Autodesk Inventor part; units mm, degrees
(part 5 of 6)
  line L1245 (-76.5118, -134.1228) -> (-98.4236, -156.0346) projected
  line L1246 (-98.4236, -156.0346) -> (-76.5118, -177.9464) projected
  line L1247 (-76.5118, -177.9464) -> (-54.6, -156.0346) projected
  line L1248 (72.9197, -181.5385) -> (51.0079, -159.6267) projected
  line L1249 (51.0079, -159.6267) -> (29.096, -181.5385) projected
  line L1250 (29.096, -181.5385) -> (51.0079, -203.4504) projected
  line L1251 (51.0079, -203.4504) -> (72.9197, -181.5385) projected
  line L1252 (-72.9197, -130.5307) -> (-51.0079, -152.4425) projected
  line L1253 (-51.0079, -152.4425) -> (-29.096, -130.5307) projected
  line L1254 (-29.096, -130.5307) -> (-51.0079, -108.6189) projected
  line L1255 (-51.0079, -108.6189) -> (-72.9197, -130.5307) projected
  line L1256 (-146.05, -222.25) -> (-146.05, -247.4846) projected
  line L1257 (-146.05, -247.4846) -> (-131.1117, -232.5464) projected
  line L1258 (-131.1117, -232.5464) -> (-146.2009, -217.4573) projected
  arc A181 (-146.05, -222.25) -> (-146.2009, -217.4573) centre (-222.25, -222.25) ccw projected
  line L1259 (-29.096, -232.5464) -> (-51.0079, -210.6346) projected
  line L1260 (-51.0079, -210.6346) -> (-72.9197, -232.5464) projected
  line L1261 (-72.9197, -232.5464) -> (-51.0079, -254.4582) projected
  line L1262 (-51.0079, -254.4582) -> (-29.096, -232.5464) projected
  line L1263 (-43.9918, -298.45) -> (-29.096, -283.5542) projected
  line L1264 (-29.096, -283.5542) -> (-51.0079, -261.6424) projected
  line L1265 (-51.0079, -261.6424) -> (-72.9197, -283.5542) projected
  line L1266 (-72.9197, -283.5542) -> (-58.0239, -298.45) projected
  line L1267 (-58.0239, -298.45) -> (-43.9918, -298.45) projected
  line L1268 (-87.8154, -298.45) -> (-65.2081, -298.45) projected
  line L1269 (-65.2081, -298.45) -> (-76.5118, -287.1463) projected
  line L1270 (-76.5118, -287.1463) -> (-87.8154, -298.45) projected
  line L1271 (80.1039, -283.5542) -> (94.9996, -298.45) projected
  line L1272 (94.9996, -298.45) -> (109.0318, -298.45) projected
  line L1273 (109.0318, -298.45) -> (123.9275, -283.5542) projected
  line L1274 (123.9275, -283.5542) -> (102.0157, -261.6424) projected
  line L1275 (102.0157, -261.6424) -> (80.1039, -283.5542) projected
  line L1276 (14.2003, -298.45) -> (36.8076, -298.45) projected
  line L1277 (36.8076, -298.45) -> (25.5039, -287.1463) projected
  line L1278 (25.5039, -287.1463) -> (14.2003, -298.45) projected
  line L1279 (80.1039, -181.5385) -> (102.0157, -203.4504) projected
  line L1280 (102.0157, -203.4504) -> (123.9275, -181.5385) projected
  line L1281 (123.9275, -181.5385) -> (102.0157, -159.6267) projected
  line L1282 (102.0157, -159.6267) -> (80.1039, -181.5385) projected
  line L1283 (225.9432, -79.5228) -> (204.0314, -57.611) projected
  line L1284 (204.0314, -57.611) -> (182.1196, -79.5228) projected
  line L1285 (182.1196, -79.5228) -> (204.0314, -101.4346) projected
  line L1286 (204.0314, -101.4346) -> (225.9432, -79.5228) projected
  line L1287 (298.45, -14.2003) -> (284.1353, -28.515) projected
  line L1288 (284.1353, -28.515) -> (298.45, -42.8297) projected
  line L1289 (298.45, -42.8297) -> (298.45, -14.2003) projected
  line L1290 (258.6314, -54.0189) -> (280.5432, -75.9307) projected
  line L1291 (280.5432, -75.9307) -> (298.45, -58.0239) projected
  line L1292 (298.45, -58.0239) -> (298.45, -50.0139) projected
  line L1293 (298.45, -50.0139) -> (280.5432, -32.1071) projected
  line L1294 (280.5432, -32.1071) -> (258.6314, -54.0189) projected
  arc A182 (222.25, -146.05) -> (217.4573, -146.2009) centre (222.25, -222.25) ccw projected
  line L1295 (222.25, -146.05) -> (241.4626, -146.05) projected
  line L1296 (241.4626, -146.05) -> (229.5353, -134.1228) projected
  line L1297 (229.5353, -134.1228) -> (217.4573, -146.2009) projected
  line L1298 (131.1117, -181.5385) -> (149.4183, -199.8451) projected
  arc A183 (165.1681, -171.7713) -> (149.4183, -199.8451) centre (222.25, -222.25) ccw projected
  line L1299 (165.1681, -171.7713) -> (153.0236, -159.6267) projected
  line L1300 (153.0236, -159.6267) -> (131.1117, -181.5385) projected
  line L1301 (7.0161, -298.45) -> (21.9118, -283.5542) projected
  line L1302 (21.9118, -283.5542) -> (0, -261.6424) projected
  line L1303 (0, -261.6424) -> (-21.9118, -283.5542) projected
  line L1304 (-21.9118, -283.5542) -> (-7.0161, -298.45) projected
  line L1305 (-7.0161, -298.45) -> (7.0161, -298.45) projected
  line L1306 (298.45, 138.8233) -> (284.1353, 124.5086) projected
  line L1307 (284.1353, 124.5086) -> (298.45, 110.1939) projected
  line L1308 (298.45, 110.1939) -> (298.45, 138.8233) projected
  line L1309 (258.6314, 99.0047) -> (280.5432, 77.0928) projected
  line L1310 (280.5432, 77.0928) -> (298.45, 94.9996) projected
  line L1311 (298.45, 94.9996) -> (298.45, 103.0097) projected
  line L1312 (298.45, 103.0097) -> (280.5432, 120.9165) projected
  line L1313 (280.5432, 120.9165) -> (258.6314, 99.0047) projected
  line L1314 (233.1274, 22.4929) -> (255.0393, 0.5811) projected
  line L1315 (255.0393, 0.5811) -> (276.9511, 22.4929) projected
  line L1316 (276.9511, 22.4929) -> (255.0393, 44.4047) projected
  line L1317 (255.0393, 44.4047) -> (233.1274, 22.4929) projected
  line L1318 (207.6235, -3.011) -> (229.5353, -24.9229) projected
  line L1319 (229.5353, -24.9229) -> (251.4472, -3.011) projected
  line L1320 (251.4472, -3.011) -> (229.5353, 18.9008) projected
  line L1321 (229.5353, 18.9008) -> (207.6235, -3.011) projected
  line L1322 (174.9354, -28.515) -> (153.0236, -6.6031) projected
  line L1323 (153.0236, -6.6031) -> (131.1117, -28.515) projected
  line L1324 (131.1117, -28.515) -> (153.0236, -50.4268) projected
  line L1325 (153.0236, -50.4268) -> (174.9354, -28.515) projected
  line L1326 (159.5933, 7.1508) -> (174.933, 22.4952) projected
  line L1327 (174.933, 22.4952) -> (153.0236, 44.4047) projected
  line L1328 (153.0236, 44.4047) -> (131.1117, 22.4929) projected
  line L1329 (131.1117, 22.4929) -> (153.0236, 0.5811) projected
  line L1330 (153.0236, 0.5811) -> (159.5933, 7.1508) projected
  line L1331 (149.4315, 47.9968) -> (127.5196, 69.9086) projected
  line L1332 (127.5196, 69.9086) -> (105.6078, 47.9968) projected
  line L1333 (105.6078, 47.9968) -> (127.5196, 26.085) projected
  line L1334 (127.5196, 26.085) -> (149.4315, 47.9968) projected
  line L1335 (156.6157, 99.0047) -> (178.5275, 77.0928) projected
  line L1336 (178.5275, 77.0928) -> (200.4393, 99.0047) projected
  line L1337 (200.4393, 99.0047) -> (178.5275, 120.9165) projected
  line L1338 (178.5275, 120.9165) -> (156.6157, 99.0047) projected
  line L1339 (80.1039, 175.5165) -> (102.0157, 153.6046) projected
  line L1340 (102.0157, 153.6046) -> (123.9275, 175.5165) projected
  line L1341 (123.9275, 175.5165) -> (102.0157, 197.4283) projected
  line L1342 (102.0157, 197.4283) -> (80.1039, 175.5165) projected
  line L1343 (0, 146.4204) -> (-21.9118, 124.5086) projected
  line L1344 (-21.9118, 124.5086) -> (0, 102.5968) projected
  line L1345 (0, 102.5968) -> (21.9118, 124.5086) projected
  line L1346 (21.9118, 124.5086) -> (0, 146.4204) projected
  line L1347 (146.05, 222.25) -> (146.05, 241.4626) projected
  line L1348 (146.05, 241.4626) -> (131.1117, 226.5243) projected
  line L1349 (131.1117, 226.5243) -> (146.9294, 210.7066) projected
  arc A184 (146.05, 222.25) -> (146.9294, 210.7066) centre (222.25, 222.25) ccw projected
  line L1350 (80.1039, -130.5307) -> (102.0157, -152.4425) projected
  line L1351 (102.0157, -152.4425) -> (123.9275, -130.5307) projected
  line L1352 (123.9275, -130.5307) -> (102.0157, -108.6189) projected
  line L1353 (102.0157, -108.6189) -> (80.1039, -130.5307) projected
  line L1354 (47.4158, -156.0346) -> (25.5039, -134.1228) projected
  line L1355 (25.5039, -134.1228) -> (3.5921, -156.0346) projected
  line L1356 (3.5921, -156.0346) -> (25.5039, -177.9464) projected
  line L1357 (25.5039, -177.9464) -> (47.4158, -156.0346) projected
  line L1358 (98.4236, 252.0282) -> (76.5118, 273.9401) projected
  line L1359 (76.5118, 273.9401) -> (54.6, 252.0282) projected
  line L1360 (54.6, 252.0282) -> (76.5118, 230.1164) projected
  line L1361 (76.5118, 230.1164) -> (98.4236, 252.0282) projected
  line L1362 (3.5921, 252.0282) -> (25.5039, 230.1164) projected
  line L1363 (25.5039, 230.1164) -> (47.4158, 252.0282) projected
  line L1364 (47.4158, 252.0282) -> (25.5039, 273.9401) projected
  line L1365 (25.5039, 273.9401) -> (3.5921, 252.0282) projected
  line L1366 (-3.5921, 252.0282) -> (-25.5039, 273.9401) projected
  line L1367 (-25.5039, 273.9401) -> (-47.4158, 252.0282) projected
  line L1368 (-47.4158, 252.0282) -> (-25.5039, 230.1164) projected
  line L1369 (-25.5039, 230.1164) -> (-3.5921, 252.0282) projected
  line L1370 (-103.0097, 298.45) -> (-123.9275, 277.5322) projected
  line L1371 (-123.9275, 277.5322) -> (-102.0157, 255.6203) projected
  line L1372 (-102.0157, 255.6203) -> (-80.1039, 277.5322) projected
  line L1373 (-80.1039, 277.5322) -> (-101.0217, 298.45) projected
  line L1374 (-101.0217, 298.45) -> (-103.0097, 298.45) projected
  line L1375 (-80.1039, 226.5243) -> (-102.0157, 248.4361) projected
  line L1376 (-102.0157, 248.4361) -> (-123.9275, 226.5243) projected
  line L1377 (-123.9275, 226.5243) -> (-102.0157, 204.6125) projected
  line L1378 (-102.0157, 204.6125) -> (-80.1039, 226.5243) projected
  line L1379 (-105.6078, 201.0204) -> (-127.5196, 222.9322) projected
  line L1380 (-127.5196, 222.9322) -> (-148.9209, 201.531) projected
  arc A185 (-149.1495, 200.7384) -> (-148.9209, 201.531) centre (-222.25, 222.25) ccw projected
  line L1381 (-149.1495, 200.7384) -> (-127.5196, 179.1086) projected
  line L1382 (-127.5196, 179.1086) -> (-105.6078, 201.0204) projected
  line L1383 (-80.1039, 175.5165) -> (-102.0157, 197.4283) projected
  line L1384 (-102.0157, 197.4283) -> (-123.9275, 175.5165) projected
  line L1385 (-123.9275, 175.5165) -> (-102.0157, 153.6046) projected
  line L1386 (-102.0157, 153.6046) -> (-80.1039, 175.5165) projected
  line L1387 (-3.5921, 150.0125) -> (-25.5039, 171.9243) projected
  line L1388 (-25.5039, 171.9243) -> (-47.4158, 150.0125) projected
  line L1389 (-47.4158, 150.0125) -> (-25.5039, 128.1007) projected
  line L1390 (-25.5039, 128.1007) -> (-3.5921, 150.0125) projected
  line L1391 (-131.1117, 124.5086) -> (-153.0236, 146.4204) projected
  line L1392 (-153.0236, 146.4204) -> (-174.9354, 124.5086) projected
  line L1393 (-174.9354, 124.5086) -> (-153.0236, 102.5968) projected
  line L1394 (-153.0236, 102.5968) -> (-131.1117, 124.5086) projected
  line L1395 (-131.1117, 73.5007) -> (-153.0236, 95.4126) projected
  line L1396 (-153.0236, 95.4126) -> (-174.9354, 73.5007) projected
  line L1397 (-174.9354, 73.5007) -> (-153.0236, 51.5889) projected
  line L1398 (-153.0236, 51.5889) -> (-131.1117, 73.5007) projected
  line L1399 (-149.4315, -54.0189) -> (-127.5196, -75.9307) projected
  line L1400 (-127.5196, -75.9307) -> (-105.6078, -54.0189) projected
  line L1401 (-105.6078, -54.0189) -> (-127.5196, -32.1071) projected
  line L1402 (-127.5196, -32.1071) -> (-149.4315, -54.0189) projected
  line L1403 (-131.1117, -79.5228) -> (-153.0236, -57.611) projected
  line L1404 (-153.0236, -57.611) -> (-174.9354, -79.5228) projected
  line L1405 (-174.9354, -79.5228) -> (-153.0236, -101.4346) projected
  line L1406 (-153.0236, -101.4346) -> (-131.1117, -79.5228) projected
  arc A186 (-222.25, 146.05) -> (-210.7066, 146.9294) centre (-222.25, 222.25) ccw projected
  line L1407 (-222.25, 146.05) -> (-247.4846, 146.05) projected
  line L1408 (-247.4846, 146.05) -> (-229.5353, 128.1007) projected
  line L1409 (-229.5353, 128.1007) -> (-210.7066, 146.9294) projected
  line L1410 (-258.6314, 99.0047) -> (-280.5432, 120.9165) projected
  line L1411 (-280.5432, 120.9165) -> (-298.45, 103.0097) projected
  line L1412 (-298.45, 103.0097) -> (-298.45, 94.9996) projected
  line L1413 (-298.45, 94.9996) -> (-280.5432, 77.0928) projected
  line L1414 (-280.5432, 77.0928) -> (-258.6314, 99.0047) projected
  line L1415 (-156.6157, 47.9968) -> (-178.5275, 69.9086) projected
  line L1416 (-178.5275, 69.9086) -> (-200.4331, 48.0031) projected
  line L1417 (-200.4331, 48.0031) -> (-178.5246, 26.0879) projected
  line L1418 (-178.5246, 26.0879) -> (-156.6157, 47.9968) projected
  line L1419 (-258.6314, 47.9968) -> (-280.5432, 69.9086) projected
  line L1420 (-280.5432, 69.9086) -> (-298.45, 52.0018) projected
  line L1421 (-298.45, 52.0018) -> (-298.45, 43.9918) projected
  line L1422 (-298.45, 43.9918) -> (-280.5432, 26.085) projected
  line L1423 (-280.5432, 26.085) -> (-258.6314, 47.9968) projected
  line L1424 (-233.1274, -28.515) -> (-255.0393, -6.6031) projected
  line L1425 (-255.0393, -6.6031) -> (-276.9511, -28.515) projected
  line L1426 (-276.9511, -28.515) -> (-255.0393, -50.4268) projected
  line L1427 (-255.0393, -50.4268) -> (-233.1274, -28.515) projected
  line L1428 (-298.45, -42.8297) -> (-284.1353, -28.515) projected
  line L1429 (-284.1353, -28.515) -> (-298.45, -14.2003) projected
  line L1430 (-298.45, -14.2003) -> (-298.45, -42.8297) projected
  line L1431 (-298.45, -93.8375) -> (-284.1353, -79.5228) projected
  line L1432 (-284.1353, -79.5228) -> (-298.45, -65.2081) projected
  line L1433 (-298.45, -65.2081) -> (-298.45, -93.8375) projected
  line L1434 (-178.5275, 18.9008) -> (-200.4393, -3.011) projected
  line L1435 (-200.4393, -3.011) -> (-178.5275, -24.9229) projected
  line L1436 (-178.5275, -24.9229) -> (-156.6157, -3.011) projected
  line L1437 (-156.6157, -3.011) -> (-178.5275, 18.9008) projected
  line L1438 (-258.6314, -3.011) -> (-280.5432, 18.9008) projected
  line L1439 (-280.5432, 18.9008) -> (-298.45, 0.994) projected
  line L1440 (-298.45, 0.994) -> (-298.45, -7.0161) projected
  line L1441 (-298.45, -7.0161) -> (-280.5432, -24.9229) projected
  line L1442 (-280.5432, -24.9229) -> (-258.6314, -3.011) projected
  line L1443 (-233.1274, 22.4929) -> (-255.0393, 44.4047) projected
  line L1444 (-255.0393, 44.4047) -> (-276.9511, 22.4929) projected
  line L1445 (-276.9511, 22.4929) -> (-255.0393, 0.5811) projected
  line L1446 (-255.0393, 0.5811) -> (-233.1274, 22.4929) projected
  line L1447 (-182.1196, 73.5007) -> (-204.0314, 95.4126) projected
  line L1448 (-204.0314, 95.4126) -> (-225.9331, 73.5109) projected
  line L1449 (-225.9331, 73.5109) -> (-204.0246, 51.5957) projected
  line L1450 (-204.0246, 51.5957) -> (-182.1196, 73.5007) projected
  line L1451 (-298.45, 110.1939) -> (-284.1353, 124.5086) projected
  line L1452 (-284.1353, 124.5086) -> (-298.45, 138.8233) projected
  line L1453 (-298.45, 138.8233) -> (-298.45, 110.1939) projected
  line L1454 (-21.9118, 175.5165) -> (0, 153.6046) projected
  line L1455 (0, 153.6046) -> (21.9118, 175.5165) projected
  line L1456 (21.9118, 175.5165) -> (0, 197.4283) projected
  line L1457 (0, 197.4283) -> (-21.9118, 175.5165) projected
  line L1458 (-105.6078, -105.0267) -> (-127.5196, -83.1149) projected
  line L1459 (-127.5196, -83.1149) -> (-149.4315, -105.0267) projected
  line L1460 (-149.4315, -105.0267) -> (-127.5196, -126.9386) projected
  line L1461 (-127.5196, -126.9386) -> (-105.6078, -105.0267) projected
  line L1462 (-153.0236, -50.4268) -> (-131.1117, -28.515) projected
  line L1463 (-131.1117, -28.515) -> (-153.0236, -6.6031) projected
  line L1464 (-153.0236, -6.6031) -> (-174.9354, -28.515) projected
  line L1465 (-174.9354, -28.515) -> (-153.0236, -50.4268) projected
  line L1466 (-156.6157, 99.0047) -> (-178.5275, 120.9165) projected
  line L1467 (-178.5275, 120.9165) -> (-200.4393, 99.0047) projected
  line L1468 (-200.4393, 99.0047) -> (-178.5275, 77.0928) projected
  line L1469 (-178.5275, 77.0928) -> (-156.6157, 99.0047) projected
  line L1470 (-105.6078, 99.0047) -> (-127.5196, 120.9165) projected
  line L1471 (-127.5196, 120.9165) -> (-149.4315, 99.0047) projected
  line L1472 (-149.4315, 99.0047) -> (-127.5196, 77.0928) projected
  line L1473 (-127.5196, 77.0928) -> (-105.6078, 99.0047) projected
  line L1474 (-29.096, 175.5165) -> (-51.0079, 197.4283) projected
  line L1475 (-51.0079, 197.4283) -> (-72.9197, 175.5165) projected
  line L1476 (-72.9197, 175.5165) -> (-51.0079, 153.6046) projected
  line L1477 (-51.0079, 153.6046) -> (-29.096, 175.5165) projected
  line L1478 (-149.4315, 150.0125) -> (-127.5196, 128.1007) projected
  line L1479 (-127.5196, 128.1007) -> (-105.6078, 150.0125) projected
  line L1480 (-105.6078, 150.0125) -> (-127.5196, 171.9243) projected
  line L1481 (-127.5196, 171.9243) -> (-149.4315, 150.0125) projected
  line L1482 (-54.6, 201.0204) -> (-76.5118, 222.9322) projected
  line L1483 (-76.5118, 222.9322) -> (-98.4236, 201.0204) projected
  line L1484 (-98.4236, 201.0204) -> (-76.5118, 179.1086) projected
  line L1485 (-76.5118, 179.1086) -> (-54.6, 201.0204) projected
  line L1486 (-105.6078, 252.0282) -> (-127.5196, 273.9401) projected
  line L1487 (-127.5196, 273.9401) -> (-146.05, 255.4097) projected
  line L1488 (-146.05, 255.4097) -> (-146.05, 248.6468) projected
  line L1489 (-146.05, 248.6468) -> (-127.5196, 230.1164) projected
  line L1490 (-127.5196, 230.1164) -> (-105.6078, 252.0282) projected
  line L1491 (-59.186, 298.45) -> (-93.8375, 298.45) projected
  line L1492 (-93.8375, 298.45) -> (-76.5118, 281.1243) projected
  line L1493 (-76.5118, 281.1243) -> (-59.186, 298.45) projected
  line L1494 (21.9118, 226.5243) -> (0, 248.4361) projected
  line L1495 (0, 248.4361) -> (-21.9118, 226.5243) projected
  line L1496 (-21.9118, 226.5243) -> (0, 204.6125) projected
  line L1497 (0, 204.6125) -> (21.9118, 226.5243) projected
  line L1498 (29.096, 226.5243) -> (51.0079, 204.6125) projected
  line L1499 (51.0079, 204.6125) -> (72.9197, 226.5243) projected
  line L1500 (72.9197, 226.5243) -> (51.0079, 248.4361) projected
  line L1501 (51.0079, 248.4361) -> (29.096, 226.5243) projected
  line L1502 (103.0097, 298.45) -> (101.0217, 298.45) projected
  line L1503 (101.0217, 298.45) -> (80.1039, 277.5322) projected
  line L1504 (80.1039, 277.5322) -> (102.0157, 255.6203) projected
  line L1505 (102.0157, 255.6203) -> (123.9275, 277.5322) projected
  line L1506 (123.9275, 277.5322) -> (103.0097, 298.45) projected
  line L1507 (29.096, -130.5307) -> (51.0079, -152.4425) projected
  line L1508 (51.0079, -152.4425) -> (72.9197, -130.5307) projected
  line L1509 (72.9197, -130.5307) -> (51.0079, -108.6189) projected
  line L1510 (51.0079, -108.6189) -> (29.096, -130.5307) projected
  line L1511 (105.6078, -105.0267) -> (127.5196, -126.9386) projected
  line L1512 (127.5196, -126.9386) -> (149.4315, -105.0267) projected
  line L1513 (149.4315, -105.0267) -> (127.5196, -83.1149) projected
  line L1514 (127.5196, -83.1149) -> (105.6078, -105.0267) projected
  arc A187 (148.9209, 201.531) -> (149.1495, 200.7384) centre (222.25, 222.25) ccw projected
  line L1515 (148.9209, 201.531) -> (127.5196, 222.9322) projected
  line L1516 (127.5196, 222.9322) -> (105.6078, 201.0204) projected
  line L1517 (105.6078, 201.0204) -> (127.5196, 179.1086) projected
  line L1518 (127.5196, 179.1086) -> (149.1495, 200.7384) projected
  line L1519 (3.5921, 150.0125) -> (25.5039, 128.1007) projected
  line L1520 (25.5039, 128.1007) -> (47.4158, 150.0125) projected
  line L1521 (47.4158, 150.0125) -> (25.5039, 171.9243) projected
  line L1522 (25.5039, 171.9243) -> (3.5921, 150.0125) projected
  line L1523 (105.6078, 150.0125) -> (127.5196, 128.1007) projected
  line L1524 (127.5196, 128.1007) -> (149.4315, 150.0125) projected
  line L1525 (149.4315, 150.0125) -> (127.5196, 171.9243) projected
  line L1526 (127.5196, 171.9243) -> (105.6078, 150.0125) projected
  line L1527 (80.1039, 124.5086) -> (102.0157, 102.5968) projected
  line L1528 (102.0157, 102.5968) -> (123.9275, 124.5086) projected
  line L1529 (123.9275, 124.5086) -> (102.0157, 146.4204) projected
  line L1530 (102.0157, 146.4204) -> (80.1039, 124.5086) projected
  line L1531 (131.1117, 73.5007) -> (153.0236, 51.5889) projected
  line L1532 (153.0236, 51.5889) -> (174.9354, 73.5007) projected
  line L1533 (174.9354, 73.5007) -> (153.0236, 95.4126) projected
  line L1534 (153.0236, 95.4126) -> (131.1117, 73.5007) projected
  line L1535 (174.9354, -79.5228) -> (153.0236, -57.611) projected
  line L1536 (153.0236, -57.611) -> (131.1117, -79.5228) projected
  line L1537 (131.1117, -79.5228) -> (153.0236, -101.4346) projected
  line L1538 (153.0236, -101.4346) -> (174.9354, -79.5228) projected
  line L1539 (200.4393, -3.011) -> (178.5275, 18.9008) projected
  line L1540 (178.5275, 18.9008) -> (156.6157, -3.011) projected
  line L1541 (156.6157, -3.011) -> (178.5275, -24.9229) projected
  line L1542 (178.5275, -24.9229) -> (200.4393, -3.011) projected
  line L1543 (156.6157, 47.9968) -> (178.5246, 26.0879) projected
  line L1544 (178.5246, 26.0879) -> (200.4331, 48.0031) projected
  line L1545 (200.4331, 48.0031) -> (178.5275, 69.9086) projected
  line L1546 (178.5275, 69.9086) -> (156.6157, 47.9968) projected
  line L1547 (258.6314, 47.9968) -> (280.5432, 26.085) projected
  line L1548 (280.5432, 26.085) -> (298.45, 43.9918) projected
  line L1549 (298.45, 43.9918) -> (298.45, 52.0018) projected
  line L1550 (298.45, 52.0018) -> (280.5432, 69.9086) projected
  line L1551 (280.5432, 69.9086) -> (258.6314, 47.9968) projected
  line L1552 (254.6689, 146.05) -> (233.1274, 124.5086) projected
  line L1553 (233.1274, 124.5086) -> (255.0247, 102.6114) projected
  line L1554 (255.0247, 102.6114) -> (276.9331, 124.5266) projected
  line L1555 (276.9331, 124.5266) -> (255.4097, 146.05) projected
  line L1556 (255.4097, 146.05) -> (254.6689, 146.05) projected
  line L1557 (298.45, 87.8154) -> (284.1353, 73.5007) projected
  line L1558 (284.1353, 73.5007) -> (298.45, 59.186) projected
  line L1559 (298.45, 59.186) -> (298.45, 87.8154) projected
  line L1560 (123.9275, -232.5464) -> (102.0157, -210.6346) projected
  line L1561 (102.0157, -210.6346) -> (80.1039, -232.5464) projected
  line L1562 (80.1039, -232.5464) -> (102.0157, -254.4582) projected
  line L1563 (102.0157, -254.4582) -> (123.9275, -232.5464) projected
  line L1564 (156.6157, -156.0346) -> (168.6598, -168.0787) projected
  arc A188 (195.3578, -150.9531) -> (168.6598, -168.0787) centre (222.25, -222.25) ccw projected
  line L1565 (195.3578, -150.9531) -> (178.5275, -134.1228) projected
  line L1566 (178.5275, -134.1228) -> (156.6157, -156.0346) projected
  line L1567 (268.616, -146.05) -> (292.4704, -146.05) projected
  line L1568 (292.4704, -146.05) -> (280.5432, -134.1228) projected
  line L1569 (280.5432, -134.1228) -> (268.616, -146.05) projected
  line L1570 (298.45, -109.0318) -> (298.45, -101.0217) projected
  line L1571 (298.45, -101.0217) -> (280.5432, -83.1149) projected
  line L1572 (280.5432, -83.1149) -> (258.6314, -105.0267) projected
  line L1573 (258.6314, -105.0267) -> (280.5432, -126.9386) projected
  line L1574 (280.5432, -126.9386) -> (298.45, -109.0318) projected
  line L1575 (258.6314, -3.011) -> (280.5432, -24.9229) projected
  line L1576 (280.5432, -24.9229) -> (298.45, -7.0161) projected
  line L1577 (298.45, -7.0161) -> (298.45, 0.994) projected
  line L1578 (298.45, 0.994) -> (280.5432, 18.9008) projected
  line L1579 (280.5432, 18.9008) -> (258.6314, -3.011) projected
  line L1580 (200.4393, -105.0267) -> (178.5275, -83.1149) projected
  line L1581 (178.5275, -83.1149) -> (156.6157, -105.0267) projected
  line L1582 (156.6157, -105.0267) -> (178.5275, -126.9386) projected
  line L1583 (178.5275, -126.9386) -> (200.4393, -105.0267) projected
  line L1584 (98.4236, -207.0425) -> (76.5118, -185.1306) projected
  line L1585 (76.5118, -185.1306) -> (54.6, -207.0425) projected
  line L1586 (54.6, -207.0425) -> (76.5118, -228.9543) projected
  line L1587 (76.5118, -228.9543) -> (98.4236, -207.0425) projected
  line L1588 (58.0239, -298.45) -> (72.9197, -283.5542) projected
  line L1589 (72.9197, -283.5542) -> (51.0079, -261.6424) projected
  line L1590 (51.0079, -261.6424) -> (29.096, -283.5542) projected
  line L1591 (29.096, -283.5542) -> (43.9918, -298.45) projected
  line L1592 (43.9918, -298.45) -> (58.0239, -298.45) projected
  line L1593 (146.05, -261.4318) -> (146.05, -254.6689) projected
  line L1594 (146.05, -254.6689) -> (127.5196, -236.1385) projected
  line L1595 (127.5196, -236.1385) -> (105.6078, -258.0503) projected
  line L1596 (105.6078, -258.0503) -> (127.5196, -279.9621) projected
  line L1597 (127.5196, -279.9621) -> (146.05, -261.4318) projected
  line L1598 (-138.8233, -298.45) -> (-116.216, -298.45) projected
  line L1599 (-116.216, -298.45) -> (-127.5196, -287.1463) projected
  line L1600 (-127.5196, -287.1463) -> (-138.8233, -298.45) projected
  line L1601 (-54.6, -207.0425) -> (-76.5118, -185.1306) projected
  line L1602 (-76.5118, -185.1306) -> (-98.4236, -207.0425) projected
  line L1603 (-98.4236, -207.0425) -> (-76.5118, -228.9543) projected
  line L1604 (-76.5118, -228.9543) -> (-54.6, -207.0425) projected
  line L1605 (-105.6078, -207.0425) -> (-127.5196, -185.1306) projected
  line L1606 (-127.5196, -185.1306) -> (-147.9092, -205.5202) projected
  arc A189 (-147.1553, -209.3187) -> (-147.9092, -205.5202) centre (-222.25, -222.25) ccw projected
  line L1607 (-147.1553, -209.3187) -> (-127.5196, -228.9543) projected
  line L1608 (-127.5196, -228.9543) -> (-105.6078, -207.0425) projected
  line L1609 (-21.9118, -130.5307) -> (0, -152.4425) projected
  line L1610 (0, -152.4425) -> (21.9118, -130.5307) projected
  line L1611 (21.9118, -130.5307) -> (0, -108.6189) projected
  line L1612 (0, -108.6189) -> (-21.9118, -130.5307) projected
  line L1613 (-21.9118, -232.5464) -> (0, -254.4582) projected
  line L1614 (0, -254.4582) -> (21.9118, -232.5464) projected
  line L1615 (21.9118, -232.5464) -> (0, -210.6346) projected
  line L1616 (0, -210.6346) -> (-21.9118, -232.5464) projected
  line L1617 (-80.1039, -130.5307) -> (-102.0157, -108.6189) projected
  line L1618 (-102.0157, -108.6189) -> (-123.9275, -130.5307) projected
  line L1619 (-123.9275, -130.5307) -> (-102.0157, -152.4425) projected
  line L1620 (-102.0157, -152.4425) -> (-80.1039, -130.5307) projected
  arc A190 (-168.6598, -168.0787) -> (-195.3578, -150.9531) centre (-222.25, -222.25) ccw projected
  line L1621 (-168.6598, -168.0787) -> (-156.6157, -156.0346) projected
  line L1622 (-156.6157, -156.0346) -> (-178.5275, -134.1228) projected
  line L1623 (-178.5275, -134.1228) -> (-195.3578, -150.9531) projected
  line L1624 (-178.5275, -75.9307) -> (-156.6157, -54.0189) projected
  line L1625 (-156.6157, -54.0189) -> (-178.5275, -32.1071) projected
  line L1626 (-178.5275, -32.1071) -> (-200.4393, -54.0189) projected
  line L1627 (-200.4393, -54.0189) -> (-178.5275, -75.9307) projected
  line L1628 (-298.45, -144.8454) -> (-284.1353, -130.5307) projected
  line L1629 (-284.1353, -130.5307) -> (-298.45, -116.216) projected
  line L1630 (-298.45, -116.216) -> (-298.45, -144.8454) projected
  line L1631 (-248.6468, -146.05) -> (-233.1274, -130.5307) projected
  line L1632 (-233.1274, -130.5307) -> (-255.0393, -108.6189) projected
  line L1633 (-255.0393, -108.6189) -> (-276.9511, -130.5307) projected
  line L1634 (-276.9511, -130.5307) -> (-261.4318, -146.05) projected
  line L1635 (-261.4318, -146.05) -> (-248.6468, -146.05) projected
  line L1636 (-229.5353, -126.9386) -> (-207.6235, -105.0267) projected
  line L1637 (-207.6235, -105.0267) -> (-229.5353, -83.1149) projected
  line L1638 (-229.5353, -83.1149) -> (-251.4472, -105.0267) projected
  line L1639 (-251.4472, -105.0267) -> (-229.5353, -126.9386) projected
  line L1640 (-200.7384, -149.1495) -> (-182.1196, -130.5307) projected
  line L1641 (-182.1196, -130.5307) -> (-204.0314, -108.6189) projected
  line L1642 (-204.0314, -108.6189) -> (-225.9432, -130.5307) projected
  line L1643 (-225.9432, -130.5307) -> (-209.3187, -147.1553) projected
  arc A191 (-200.7384, -149.1495) -> (-209.3187, -147.1553) centre (-222.25, -222.25) ccw projected
  line L1644 (-105.6078, -156.0346) -> (-127.5196, -134.1228) projected
  line L1645 (-127.5196, -134.1228) -> (-149.4315, -156.0346) projected
  line L1646 (-149.4315, -156.0346) -> (-127.5196, -177.9464) projected
  line L1647 (-127.5196, -177.9464) -> (-105.6078, -156.0346) projected
  line L1648 (-29.096, -181.5385) -> (-51.0079, -159.6267) projected
  line L1649 (-51.0079, -159.6267) -> (-72.9197, -181.5385) projected
  line L1650 (-72.9197, -181.5385) -> (-51.0079, -203.4504) projected
  line L1651 (-51.0079, -203.4504) -> (-29.096, -181.5385) projected
  line L1652 (3.5921, -207.0425) -> (25.5039, -228.9543) projected
  line L1653 (25.5039, -228.9543) -> (47.4158, -207.0425) projected
  line L1654 (47.4158, -207.0425) -> (25.5039, -185.1306) projected
  line L1655 (25.5039, -185.1306) -> (3.5921, -207.0425) projected
  line L1656 (-47.4158, -156.0346) -> (-25.5039, -177.9464) projected
  line L1657 (-25.5039, -177.9464) -> (-3.5921, -156.0346) projected
  line L1658 (-3.5921, -156.0346) -> (-25.5039, -134.1228) projected
  line L1659 (-25.5039, -134.1228) -> (-47.4158, -156.0346) projected
  line L1660 (-146.05, -254.6689) -> (-146.05, -261.4318) projected
  line L1661 (-146.05, -261.4318) -> (-127.5196, -279.9621) projected
  line L1662 (-127.5196, -279.9621) -> (-105.6078, -258.0503) projected
  line L1663 (-105.6078, -258.0503) -> (-127.5196, -236.1385) projected
  line L1664 (-127.5196, -236.1385) -> (-146.05, -254.6689) projected
  line L1665 (-54.6, -258.0503) -> (-76.5118, -236.1385) projected
  line L1666 (-76.5118, -236.1385) -> (-98.4236, -258.0503) projected
  line L1667 (-98.4236, -258.0503) -> (-76.5118, -279.9621) projected
  line L1668 (-76.5118, -279.9621) -> (-54.6, -258.0503) projected
  line L1669 (-123.9275, -283.5542) -> (-109.0318, -298.45) projected
  line L1670 (-109.0318, -298.45) -> (-94.9996, -298.45) projected
  line L1671 (-94.9996, -298.45) -> (-80.1039, -283.5542) projected
  line L1672 (-80.1039, -283.5542) -> (-102.0157, -261.6424) projected
  line L1673 (-102.0157, -261.6424) -> (-123.9275, -283.5542) projected
  line L1674 (146.05, -298.45) -> (146.05, -268.616) projected
  line L1675 (146.05, -268.616) -> (131.1117, -283.5542) projected
  line L1676 (131.1117, -283.5542) -> (146.0075, -298.45) projected
  line L1677 (146.0075, -298.45) -> (146.05, -298.45) projected
  line L1678 (54.6, -258.0503) -> (76.5118, -279.9621) projected
  line L1679 (76.5118, -279.9621) -> (98.4236, -258.0503) projected
  line L1680 (98.4236, -258.0503) -> (76.5118, -236.1385) projected
  line L1681 (76.5118, -236.1385) -> (54.6, -258.0503) projected
  line L1682 (47.4158, -258.0503) -> (25.5039, -236.1385) projected
  line L1683 (25.5039, -236.1385) -> (3.5921, -258.0503) projected
  line L1684 (3.5921, -258.0503) -> (25.5039, -279.9621) projected
  line L1685 (25.5039, -279.9621) -> (47.4158, -258.0503) projected
  line L1686 (105.6078, -156.0346) -> (127.5196, -177.9464) projected
  line L1687 (127.5196, -177.9464) -> (149.4315, -156.0346) projected
  line L1688 (149.4315, -156.0346) -> (127.5196, -134.1228) projected
  line L1689 (127.5196, -134.1228) -> (105.6078, -156.0346) projected
  line L1690 (251.4472, -54.0189) -> (229.5353, -32.1071) projected
  line L1691 (229.5353, -32.1071) -> (207.6235, -54.0189) projected
  line L1692 (207.6235, -54.0189) -> (229.5353, -75.9307) projected
  line L1693 (229.5353, -75.9307) -> (251.4472, -54.0189) projected
  line L1694 (298.45, -65.2081) -> (284.1353, -79.5228) projected
  line L1695 (284.1353, -79.5228) -> (298.45, -93.8375) projected
  line L1696 (298.45, -93.8375) -> (298.45, -65.2081) projected
  line L1697 (261.4318, -146.05) -> (276.9511, -130.5307) projected
  line L1698 (276.9511, -130.5307) -> (255.0393, -108.6189) projected
  line L1699 (255.0393, -108.6189) -> (233.1274, -130.5307) projected
  line L1700 (233.1274, -130.5307) -> (248.6468, -146.05) projected
  line L1701 (248.6468, -146.05) -> (261.4318, -146.05) projected
  line L1702 (251.4472, -105.0267) -> (229.5353, -83.1149) projected
  line L1703 (229.5353, -83.1149) -> (207.6235, -105.0267) projected
  line L1704 (207.6235, -105.0267) -> (229.5353, -126.9386) projected
  line L1705 (229.5353, -126.9386) -> (251.4472, -105.0267) projected
  arc A192 (146.2009, -217.4573) -> (146.05, -222.25) centre (222.25, -222.25) ccw projected
  line L1706 (146.2009, -217.4573) -> (131.1117, -232.5464) projected
  line L1707 (131.1117, -232.5464) -> (146.05, -247.4846) projected
  line L1708 (146.05, -247.4846) -> (146.05, -222.25) projected
  line L1709 (-36.8076, -298.45) -> (-14.2003, -298.45) projected
  line L1710 (-14.2003, -298.45) -> (-25.5039, -287.1463) projected
  line L1711 (-25.5039, -287.1463) -> (-36.8076, -298.45) projected
  line L1712 (298.45, 146.05) -> (262.5939, 146.05) projected
  line L1713 (262.5939, 146.05) -> (280.5247, 128.1192) projected
  line L1714 (280.5247, 128.1192) -> (298.45, 146.05) projected
  line L1715 (207.6235, 99.0047) -> (229.5246, 77.1035) projected
  line L1716 (229.5246, 77.1035) -> (251.4331, 99.0187) projected
  line L1717 (251.4331, 99.0187) -> (229.5353, 120.9165) projected
  line L1718 (229.5353, 120.9165) -> (207.6235, 99.0047) projected
  line L1719 (207.6235, 47.9968) -> (229.5353, 26.085) projected
  line L1720 (229.5353, 26.085) -> (251.4472, 47.9968) projected
  line L1721 (251.4472, 47.9968) -> (229.5353, 69.9086) projected
  line L1722 (229.5353, 69.9086) -> (207.6235, 47.9968) projected
  line L1723 (225.9432, -28.515) -> (204.0314, -6.6031) projected
  line L1724 (204.0314, -6.6031) -> (182.1196, -28.515) projected
  line L1725 (182.1196, -28.515) -> (204.0314, -50.4268) projected
  line L1726 (204.0314, -50.4268) -> (225.9432, -28.515) projected
  line L1727 (149.4315, -54.0189) -> (127.5196, -32.1071) projected
  line L1728 (127.5196, -32.1071) -> (105.6078, -54.0189) projected
  line L1729 (105.6078, -54.0189) -> (127.5196, -75.9307) projected
  line L1730 (127.5196, -75.9307) -> (149.4315, -54.0189) projected
  line L1731 (149.4315, -3.011) -> (127.5196, 18.9008) projected
  line L1732 (127.5196, 18.9008) -> (105.6078, -3.011) projected
  line L1733 (105.6078, -3.011) -> (127.5196, -24.9229) projected
  line L1734 (127.5196, -24.9229) -> (149.4315, -3.011) projected
  line L1735 (182.1196, 124.5086) -> (204.0314, 102.5968) projected
  line L1736 (204.0314, 102.5968) -> (225.9432, 124.5086) projected
  line L1737 (225.9432, 124.5086) -> (204.0314, 146.4204) projected
  line L1738 (204.0314, 146.4204) -> (182.1196, 124.5086) projected
  line L1739 (72.9197, 124.5086) -> (51.0079, 146.4204) projected
  line L1740 (51.0079, 146.4204) -> (29.096, 124.5086) projected
  line L1741 (29.096, 124.5086) -> (51.0079, 102.5968) projected
  line L1742 (51.0079, 102.5968) -> (72.9197, 124.5086) projected
  arc A193 (171.7713, 165.1681) -> (199.8451, 149.4183) centre (222.25, 222.25) ccw projected
  line L1743 (171.7713, 165.1681) -> (156.6157, 150.0125) projected
  line L1744 (156.6157, 150.0125) -> (178.5275, 128.1007) projected
  line L1745 (178.5275, 128.1007) -> (199.8451, 149.4183) projected
  line L1746 (54.6, 150.0125) -> (76.5118, 128.1007) projected
  line L1747 (76.5118, 128.1007) -> (98.4236, 150.0125) projected
  line L1748 (98.4236, 150.0125) -> (76.5118, 171.9243) projected
  line L1749 (76.5118, 171.9243) -> (54.6, 150.0125) projected
  line L1750 (76.5118, 222.9322) -> (54.6, 201.0204) projected
  line L1751 (54.6, 201.0204) -> (76.5118, 179.1086) projected
  line L1752 (76.5118, 179.1086) -> (98.4236, 201.0204) projected
  line L1753 (98.4236, 201.0204) -> (76.5118, 222.9322) projected
  line L1754 (127.5196, 273.9401) -> (105.6078, 252.0282) projected
  line L1755 (105.6078, 252.0282) -> (127.5196, 230.1164) projected
  line L1756 (127.5196, 230.1164) -> (146.05, 248.6468) projected
  line L1757 (146.05, 248.6468) -> (146.05, 255.4097) projected
  line L1758 (146.05, 255.4097) -> (127.5196, 273.9401) projected
  line L1759 (146.05, 292.4704) -> (131.1117, 277.5322) projected
  line L1760 (131.1117, 277.5322) -> (146.05, 262.5939) projected
  line L1761 (146.05, 262.5939) -> (146.05, 292.4704) projected
  line L1762 (72.9197, 277.5322) -> (52.0018, 298.45) projected
  line L1763 (52.0018, 298.45) -> (50.0139, 298.45) projected
  line L1764 (50.0139, 298.45) -> (29.096, 277.5322) projected
  line L1765 (29.096, 277.5322) -> (51.0079, 255.6203) projected
  line L1766 (51.0079, 255.6203) -> (72.9197, 277.5322) projected
  line L1767 (-0.994, 298.45) -> (-21.9118, 277.5322) projected
  line L1768 (-21.9118, 277.5322) -> (0, 255.6203) projected
  line L1769 (0, 255.6203) -> (21.9118, 277.5322) projected
  line L1770 (21.9118, 277.5322) -> (0.994, 298.45) projected
  line L1771 (0.994, 298.45) -> (-0.994, 298.45) projected
  line L1772 (-8.1782, 298.45) -> (-42.8297, 298.45) projected
  line L1773 (-42.8297, 298.45) -> (-25.5039, 281.1243) projected
  line L1774 (-25.5039, 281.1243) -> (-8.1782, 298.45) projected
  line L1775 (-110.1939, 298.45) -> (-144.8454, 298.45) projected
  line L1776 (-144.8454, 298.45) -> (-127.5196, 281.1243) projected
  line L1777 (-127.5196, 281.1243) -> (-110.1939, 298.45) projected
  line L1778 (-98.4236, 252.0282) -> (-76.5118, 230.1164) projected
  line L1779 (-76.5118, 230.1164) -> (-54.6, 252.0282) projected
  line L1780 (-54.6, 252.0282) -> (-76.5118, 273.9401) projected
  line L1781 (-76.5118, 273.9401) -> (-98.4236, 252.0282) projected
  arc A194 (-146.9294, 210.7066) -> (-146.05, 222.25) centre (-222.25, 222.25) ccw projected
  line L1782 (-146.9294, 210.7066) -> (-131.1117, 226.5243) projected
  line L1783 (-131.1117, 226.5243) -> (-146.05, 241.4626) projected
  line L1784 (-146.05, 241.4626) -> (-146.05, 222.25) projected
  line L1785 (-123.9275, 124.5086) -> (-102.0157, 102.5968) projected
  line L1786 (-102.0157, 102.5968) -> (-80.1039, 124.5086) projected
  line L1787 (-80.1039, 124.5086) -> (-102.0157, 146.4204) projected
  line L1788 (-102.0157, 146.4204) -> (-123.9275, 124.5086) projected
  line L1789 (-51.0079, 146.4204) -> (-72.9197, 124.5086) projected
  line L1790 (-72.9197, 124.5086) -> (-51.0079, 102.5968) projected
  line L1791 (-51.0079, 102.5968) -> (-29.096, 124.5086) projected
  line L1792 (-29.096, 124.5086) -> (-51.0079, 146.4204) projected
  line L1793 (-156.6157, 150.0125) -> (-171.7713, 165.1681) projected
  arc A195 (-199.8451, 149.4183) -> (-171.7713, 165.1681) centre (-222.25, 222.25) ccw projected
  line L1794 (-199.8451, 149.4183) -> (-178.5275, 128.1007) projected
  line L1795 (-178.5275, 128.1007) -> (-156.6157, 150.0125) projected
  line L1796 (-127.5196, 69.9086) -> (-149.4315, 47.9968) projected
  line L1797 (-149.4315, 47.9968) -> (-127.5196, 26.085) projected
  line L1798 (-127.5196, 26.085) -> (-105.6078, 47.9968) projected
  line L1799 (-105.6078, 47.9968) -> (-127.5196, 69.9086) projected
  line L1800 (-127.5196, -24.9229) -> (-105.6078, -3.011) projected
  line L1801 (-105.6078, -3.011) -> (-127.5196, 18.9008) projected
  line L1802 (-127.5196, 18.9008) -> (-149.4315, -3.011) projected
  line L1803 (-149.4315, -3.011) -> (-127.5196, -24.9229) projected
  line L1804 (-47.4158, 201.0204) -> (-25.5039, 179.1086) projected
  line L1805 (-25.5039, 179.1086) -> (-3.5921, 201.0204) projected
  line L1806 (-3.5921, 201.0204) -> (-25.5039, 222.9322) projected
  line L1807 (-25.5039, 222.9322) -> (-47.4158, 201.0204) projected
  line L1808 (-233.1274, 124.5086) -> (-254.6689, 146.05) projected
  line L1809 (-254.6689, 146.05) -> (-255.4097, 146.05) projected
  line L1810 (-255.4097, 146.05) -> (-276.9331, 124.5266) projected
  line L1811 (-276.9331, 124.5266) -> (-255.0247, 102.6114) projected
  line L1812 (-255.0247, 102.6114) -> (-233.1274, 124.5086) projected
  line L1813 (-233.1274, 73.5007) -> (-255.0393, 95.4126) projected
  line L1814 (-255.0393, 95.4126) -> (-276.9511, 73.5007) projected
  line L1815 (-276.9511, 73.5007) -> (-255.0393, 51.5889) projected
  line L1816 (-255.0393, 51.5889) -> (-233.1274, 73.5007) projected
  line L1817 (-182.1196, 22.4929) -> (-204.0314, 44.4047) projected
  line L1818 (-204.0314, 44.4047) -> (-225.9432, 22.4929) projected
  line L1819 (-225.9432, 22.4929) -> (-204.0314, 0.5811) projected
  line L1820 (-204.0314, 0.5811) -> (-182.1196, 22.4929) projected
  line L1821 (-298.45, 59.186) -> (-284.1353, 73.5007) projected
  line L1822 (-284.1353, 73.5007) -> (-298.45, 87.8154) projected
  line L1823 (-298.45, 87.8154) -> (-298.45, 59.186) projected
  line L1824 (-207.6235, -3.011) -> (-229.5353, 18.9008) projected
  line L1825 (-229.5353, 18.9008) -> (-251.4472, -3.011) projected
  line L1826 (-251.4472, -3.011) -> (-229.5353, -24.9229) projected
  line L1827 (-229.5353, -24.9229) -> (-207.6235, -3.011) projected
  line L1828 (-229.5353, -32.1071) -> (-251.4472, -54.0189) projected
  line L1829 (-251.4472, -54.0189) -> (-229.5353, -75.9307) projected
  line L1830 (-229.5353, -75.9307) -> (-207.6235, -54.0189) projected
  line L1831 (-207.6235, -54.0189) -> (-229.5353, -32.1071) projected
  line L1832 (-258.6314, -54.0189) -> (-280.5432, -32.1071) projected
  line L1833 (-280.5432, -32.1071) -> (-298.45, -50.0139) projected
  line L1834 (-298.45, -50.0139) -> (-298.45, -58.0239) projected
  line L1835 (-298.45, -58.0239) -> (-280.5432, -75.9307) projected
  line L1836 (-280.5432, -75.9307) -> (-258.6314, -54.0189) projected
  line L1837 (-204.0314, -6.6031) -> (-225.9432, -28.515) projected
  line L1838 (-225.9432, -28.515) -> (-204.0314, -50.4268) projected
  line L1839 (-204.0314, -50.4268) -> (-182.1196, -28.515) projected
  line L1840 (-182.1196, -28.515) -> (-204.0314, -6.6031) projected
  line L1841 (-298.45, 8.1782) -> (-284.1353, 22.4929) projected
  line L1842 (-284.1353, 22.4929) -> (-298.45, 36.8076) projected
  line L1843 (-298.45, 36.8076) -> (-298.45, 8.1782) projected
  line L1844 (-207.6235, 47.9968) -> (-229.5353, 69.9086) projected
  line L1845 (-229.5353, 69.9086) -> (-251.4472, 47.9968) projected
  line L1846 (-251.4472, 47.9968) -> (-229.5353, 26.085) projected
  line L1847 (-229.5353, 26.085) -> (-207.6235, 47.9968) projected
  line L1848 (-207.6235, 99.0047) -> (-229.5353, 120.9165) projected
  line L1849 (-229.5353, 120.9165) -> (-251.4331, 99.0187) projected
  line L1850 (-251.4331, 99.0187) -> (-229.5246, 77.1035) projected
  line L1851 (-229.5246, 77.1035) -> (-207.6235, 99.0047) projected
  line L1852 (-262.5939, 146.05) -> (-298.45, 146.05) projected
  line L1853 (-298.45, 146.05) -> (-280.5247, 128.1192) projected
  line L1854 (-280.5247, 128.1192) -> (-262.5939, 146.05) projected
  line L1855 (25.5039, 222.9322) -> (3.5921, 201.0204) projected
  line L1856 (3.5921, 201.0204) -> (25.5039, 179.1086) projected
  line L1857 (25.5039, 179.1086) -> (47.4158, 201.0204) projected
  line L1858 (47.4158, 201.0204) -> (25.5039, 222.9322) projected
  line L1859 (-131.1117, 22.4929) -> (-153.0236, 44.4047) projected
  line L1860 (-153.0236, 44.4047) -> (-174.933, 22.4952) projected
  line L1861 (-174.933, 22.4952) -> (-159.5933, 7.1508) projected
  line L1862 (-159.5933, 7.1508) -> (-153.0236, 0.5811) projected
  line L1863 (-153.0236, 0.5811) -> (-131.1117, 22.4929) projected
  line L1864 (-182.1196, 124.5086) -> (-204.0314, 146.4204) projected
  line L1865 (-204.0314, 146.4204) -> (-225.9432, 124.5086) projected
  line L1866 (-225.9432, 124.5086) -> (-204.0314, 102.5968) projected
  line L1867 (-204.0314, 102.5968) -> (-182.1196, 124.5086) projected
  line L1868 (-54.6, 150.0125) -> (-76.5118, 171.9243) projected
  line L1869 (-76.5118, 171.9243) -> (-98.4236, 150.0125) projected
  line L1870 (-98.4236, 150.0125) -> (-76.5118, 128.1007) projected
  line L1871 (-76.5118, 128.1007) -> (-54.6, 150.0125) projected
  line L1872 (-168.0787, 168.6598) -> (-153.0236, 153.6046) projected
  line L1873 (-153.0236, 153.6046) -> (-131.1117, 175.5165) projected
  line L1874 (-131.1117, 175.5165) -> (-150.9531, 195.3578) projected
  arc A196 (-168.0787, 168.6598) -> (-150.9531, 195.3578) centre (-222.25, 222.25) ccw projected
  line L1875 (-72.9197, 226.5243) -> (-51.0079, 204.6125) projected
  line L1876 (-51.0079, 204.6125) -> (-29.096, 226.5243) projected
  line L1877 (-29.096, 226.5243) -> (-51.0079, 248.4361) projected
  line L1878 (-51.0079, 248.4361) -> (-72.9197, 226.5243) projected
  line L1879 (-146.05, 262.5939) -> (-131.1117, 277.5322) projected
  line L1880 (-131.1117, 277.5322) -> (-146.05, 292.4704) projected
  line L1881 (-146.05, 292.4704) -> (-146.05, 262.5939) projected
  line L1882 (-29.096, 277.5322) -> (-50.0139, 298.45) projected
  line L1883 (-50.0139, 298.45) -> (-52.0018, 298.45) projected
  line L1884 (-52.0018, 298.45) -> (-72.9197, 277.5322) projected
  line L1885 (-72.9197, 277.5322) -> (-51.0079, 255.6203) projected
  line L1886 (-51.0079, 255.6203) -> (-29.096, 277.5322) projected
  line L1887 (42.8297, 298.45) -> (8.1782, 298.45) projected
  line L1888 (8.1782, 298.45) -> (25.5039, 281.1243) projected
  line L1889 (25.5039, 281.1243) -> (42.8297, 298.45) projected
  line L1890 (93.8375, 298.45) -> (59.186, 298.45) projected
  line L1891 (59.186, 298.45) -> (76.5118, 281.1243) projected
  line L1892 (76.5118, 281.1243) -> (93.8375, 298.45) projected
  line L1893 (144.8454, 298.45) -> (110.1939, 298.45) projected
  line L1894 (110.1939, 298.45) -> (127.5196, 281.1243) projected
  line L1895 (127.5196, 281.1243) -> (144.8454, 298.45) projected
  line L1896 (54.6, -156.0346) -> (76.5118, -177.9464) projected
  line L1897 (76.5118, -177.9464) -> (98.4236, -156.0346) projected
  line L1898 (98.4236, -156.0346) -> (76.5118, -134.1228) projected
  line L1899 (76.5118, -134.1228) -> (54.6, -156.0346) projected
  line L1900 (123.9275, 226.5243) -> (102.0157, 248.4361) projected
  line L1901 (102.0157, 248.4361) -> (80.1039, 226.5243) projected
  line L1902 (80.1039, 226.5243) -> (102.0157, 204.6125) projected
  line L1903 (102.0157, 204.6125) -> (123.9275, 226.5243) projected
  line L1904 (51.0079, 197.4283) -> (29.096, 175.5165) projected
  line L1905 (29.096, 175.5165) -> (51.0079, 153.6046) projected
  line L1906 (51.0079, 153.6046) -> (72.9197, 175.5165) projected
  line L1907 (72.9197, 175.5165) -> (51.0079, 197.4283) projected
  arc A197 (150.9531, 195.3578) -> (168.0787, 168.6598) centre (222.25, 222.25) ccw projected
  line L1908 (150.9531, 195.3578) -> (131.1117, 175.5165) projected
  line L1909 (131.1117, 175.5165) -> (153.0236, 153.6046) projected
  line L1910 (153.0236, 153.6046) -> (168.0787, 168.6598) projected
  line L1911 (131.1117, 124.5086) -> (153.0236, 102.5968) projected
  line L1912 (153.0236, 102.5968) -> (174.9354, 124.5086) projected
  line L1913 (174.9354, 124.5086) -> (153.0236, 146.4204) projected
  line L1914 (153.0236, 146.4204) -> (131.1117, 124.5086) projected
  line L1915 (105.6078, 99.0047) -> (127.5196, 77.0928) projected
  line L1916 (127.5196, 77.0928) -> (149.4315, 99.0047) projected
  line L1917 (149.4315, 99.0047) -> (127.5196, 120.9165) projected
  line L1918 (127.5196, 120.9165) -> (105.6078, 99.0047) projected
  line L1919 (200.4393, -54.0189) -> (178.5275, -32.1071) projected
  line L1920 (178.5275, -32.1071) -> (156.6157, -54.0189) projected
  line L1921 (156.6157, -54.0189) -> (178.5275, -75.9307) projected
  line L1922 (178.5275, -75.9307) -> (200.4393, -54.0189) projected
  line L1923 (182.1196, 22.4929) -> (204.0314, 0.5811) projected
  line L1924 (204.0314, 0.5811) -> (225.9432, 22.4929) projected
  line L1925 (225.9432, 22.4929) -> (204.0314, 44.4047) projected
  line L1926 (204.0314, 44.4047) -> (182.1196, 22.4929) projected
  line L1927 (182.1196, 73.5007) -> (204.0246, 51.5957) projected
  line L1928 (204.0246, 51.5957) -> (225.9331, 73.5109) projected
  line L1929 (225.9331, 73.5109) -> (204.0314, 95.4126) projected
  line L1930 (204.0314, 95.4126) -> (182.1196, 73.5007) projected
  line L1931 (233.1274, 73.5007) -> (255.0393, 51.5889) projected
  line L1932 (255.0393, 51.5889) -> (276.9511, 73.5007) projected
  line L1933 (276.9511, 73.5007) -> (255.0393, 95.4126) projected
  line L1934 (255.0393, 95.4126) -> (233.1274, 73.5007) projected
  line L1935 (247.4846, 146.05) -> (222.25, 146.05) projected
  arc A198 (210.7066, 146.9294) -> (222.25, 146.05) centre (222.25, 222.25) ccw projected
  line L1936 (210.7066, 146.9294) -> (229.5353, 128.1007) projected
  line L1937 (229.5353, 128.1007) -> (247.4846, 146.05) projected
  line L1938 (298.45, 36.8076) -> (284.1353, 22.4929) projected
  line L1939 (284.1353, 22.4929) -> (298.45, 8.1782) projected
  line L1940 (298.45, 8.1782) -> (298.45, 36.8076) projected
  line L1941 (105.6078, -207.0425) -> (127.5196, -228.9543) projected
  line L1942 (127.5196, -228.9543) -> (147.1553, -209.3187) projected
  arc A199 (147.9092, -205.5202) -> (147.1553, -209.3187) centre (222.25, -222.25) ccw projected
  line L1943 (147.9092, -205.5202) -> (127.5196, -185.1306) projected
  line L1944 (127.5196, -185.1306) -> (105.6078, -207.0425) projected
  line L1945 (209.3187, -147.1553) -> (225.9432, -130.5307) projected
  line L1946 (225.9432, -130.5307) -> (204.0314, -108.6189) projected
  line L1947 (204.0314, -108.6189) -> (182.1196, -130.5307) projected
  line L1948 (182.1196, -130.5307) -> (200.7384, -149.1495) projected
  arc A200 (209.3187, -147.1553) -> (200.7384, -149.1495) centre (222.25, -222.25) ccw projected
  line L1949 (276.9511, -79.5228) -> (255.0393, -57.611) projected
  line L1950 (255.0393, -57.611) -> (233.1274, -79.5228) projected
  line L1951 (233.1274, -79.5228) -> (255.0393, -101.4346) projected
  line L1952 (255.0393, -101.4346) -> (276.9511, -79.5228) projected
  line L1953 (298.45, -116.216) -> (284.1353, -130.5307) projected
  line L1954 (284.1353, -130.5307) -> (298.45, -144.8454) projected
  line L1955 (298.45, -144.8454) -> (298.45, -116.216) projected
  line L1956 (233.1274, -28.515) -> (255.0393, -50.4268) projected
  line L1957 (255.0393, -50.4268) -> (276.9511, -28.515) projected
  line L1958 (276.9511, -28.515) -> (255.0393, -6.6031) projected
  line L1959 (255.0393, -6.6031) -> (233.1274, -28.515) projected
  line L1960 (131.1117, -130.5307) -> (153.0236, -152.4425) projected
  line L1961 (153.0236, -152.4425) -> (174.9354, -130.5307) projected
  line L1962 (174.9354, -130.5307) -> (153.0236, -108.6189) projected
  line L1963 (153.0236, -108.6189) -> (131.1117, -130.5307) projected
  line L1964 (29.096, -232.5464) -> (51.0079, -254.4582) projected
  line L1965 (51.0079, -254.4582) -> (72.9197, -232.5464) projected
  line L1966 (72.9197, -232.5464) -> (51.0079, -210.6346) projected
  line L1967 (51.0079, -210.6346) -> (29.096, -232.5464) projected
  line L1968 (65.2081, -298.45) -> (87.8154, -298.45) projected
  line L1969 (87.8154, -298.45) -> (76.5118, -287.1463) projected
  line L1970 (76.5118, -287.1463) -> (65.2081, -298.45) projected
  line L1971 (116.216, -298.45) -> (138.8233, -298.45) projected
  line L1972 (138.8233, -298.45) -> (127.5196, -287.1463) projected
  line L1973 (127.5196, -287.1463) -> (116.216, -298.45) projected
  line L1974 (-146.05, -298.45) -> (-146.0075, -298.45) projected
  line L1975 (-146.0075, -298.45) -> (-131.1117, -283.5542) projected
  line L1976 (-131.1117, -283.5542) -> (-146.05, -268.616) projected
  line L1977 (-146.05, -268.616) -> (-146.05, -298.45) projected
  line L1978 (-3.5921, -258.0503) -> (-25.5039, -236.1385) projected
  line L1979 (-25.5039, -236.1385) -> (-47.4158, -258.0503) projected
  line L1980 (-47.4158, -258.0503) -> (-25.5039, -279.9621) projected
  line L1981 (-25.5039, -279.9621) -> (-3.5921, -258.0503) projected
  line L1982 (-80.1039, -232.5464) -> (-102.0157, -210.6346) projected
  line L1983 (-102.0157, -210.6346) -> (-123.9275, -232.5464) projected
  line L1984 (-123.9275, -232.5464) -> (-102.0157, -254.4582) projected
  line L1985 (-102.0157, -254.4582) -> (-80.1039, -232.5464) projected
  line L1986 (-80.1039, -181.5385) -> (-102.0157, -159.6267) projected
  line L1987 (-102.0157, -159.6267) -> (-123.9275, -181.5385) projected
  line L1988 (-123.9275, -181.5385) -> (-102.0157, -203.4504) projected
  line L1989 (-102.0157, -203.4504) -> (-80.1039, -181.5385) projected
  line L1990 (-21.9118, -181.5385) -> (0, -203.4504) projected
  line L1991 (0, -203.4504) -> (21.9118, -181.5385) projected
  line L1992 (21.9118, -181.5385) -> (0, -159.6267) projected
  line L1993 (0, -159.6267) -> (-21.9118, -181.5385) projected
  line L1994 (-3.5921, -207.0425) -> (-25.5039, -185.1306) projected
  line L1995 (-25.5039, -185.1306) -> (-47.4158, -207.0425) projected
  line L1996 (-47.4158, -207.0425) -> (-25.5039, -228.9543) projected
  line L1997 (-25.5039, -228.9543) -> (-3.5921, -207.0425) projected
  arc A201 (-149.4183, -199.8451) -> (-165.1681, -171.7713) centre (-222.25, -222.25) ccw projected
  line L1998 (-149.4183, -199.8451) -> (-131.1117, -181.5385) projected
  line L1999 (-131.1117, -181.5385) -> (-153.0236, -159.6267) projected
  line L2000 (-153.0236, -159.6267) -> (-165.1681, -171.7713) projected
  line L2001 (-241.4626, -146.05) -> (-222.25, -146.05) projected
  arc A202 (-217.4573, -146.2009) -> (-222.25, -146.05) centre (-222.25, -222.25) ccw projected
  line L2002 (-217.4573, -146.2009) -> (-229.5353, -134.1228) projected
  line L2003 (-229.5353, -134.1228) -> (-241.4626, -146.05) projected
  line L2004 (-204.0314, -101.4346) -> (-182.1196, -79.5228) projected
  line L2005 (-182.1196, -79.5228) -> (-204.0314, -57.611) projected
  line L2006 (-204.0314, -57.611) -> (-225.9432, -79.5228) projected
  line L2007 (-225.9432, -79.5228) -> (-204.0314, -101.4346) projected
  line L2008 (-292.4704, -146.05) -> (-268.616, -146.05) projected
  line L2009 (-268.616, -146.05) -> (-280.5432, -134.1228) projected
  line L2010 (-280.5432, -134.1228) -> (-292.4704, -146.05) projected
  line L2011 (-42.2297, 93.8186) -> (-8.7782, 93.8186) projected
  line L2012 (-8.7782, 93.8186) -> (-3.5921, 99.0047) projected
  line L2013 (-3.5921, 99.0047) -> (-25.5039, 120.9165) projected
  line L2014 (-25.5039, 120.9165) -> (-47.4158, 99.0047) projected
  line L2015 (-47.4158, 99.0047) -> (-42.2297, 93.8186) projected
  line L2016 (-52.6018, 93.8186) -> (-49.4139, 93.8186) projected
  line L2017 (-49.4139, 93.8186) -> (-51.0079, 95.4126) projected
  line L2018 (-51.0079, 95.4126) -> (-52.6018, 93.8186) projected
  arc A203 (-81.1911, 93.8186) -> (-87.7843, 88.3654) centre (-81.1911, 87.1062) ccw projected
  line L2019 (-81.1911, 93.8186) -> (-59.7861, 93.8186) projected
  line L2020 (-59.7861, 93.8186) -> (-54.6, 99.0047) projected
  line L2021 (-54.6, 99.0047) -> (-76.5118, 120.9165) projected
  line L2022 (-76.5118, 120.9165) -> (-98.4236, 99.0047) projected
  line L2023 (-98.4236, 99.0047) -> (-87.7843, 88.3654) projected
  line L2024 (-94.8078, 44.381) -> (-94.8078, 48.2458) projected
  arc A204 (-88.0954, 54.9582) -> (-94.8078, 48.2458) centre (-88.0954, 48.2458) ccw projected
  line L2025 (-88.0954, 54.9582) -> (-87.9035, 54.9582) projected
  line L2026 (-87.9035, 54.9582) -> (-87.9035, 58.5169) projected
  line L2027 (-87.9035, 58.5169) -> (-98.4236, 47.9968) projected
  line L2028 (-98.4236, 47.9968) -> (-94.8078, 44.381) projected
  line L2029 (-94.8078, 7.789) -> (-94.8078, 37.1968) projected
  line L2030 (-94.8078, 37.1968) -> (-102.0157, 44.4047) projected
  line L2031 (-102.0157, 44.4047) -> (-123.9275, 22.4929) projected
  line L2032 (-123.9275, 22.4929) -> (-102.0157, 0.5811) projected
  line L2033 (-102.0157, 0.5811) -> (-94.8078, 7.789) projected
  line L2034 (-94.8078, -43.2189) -> (-94.8078, -13.8111) projected
  line L2035 (-94.8078, -13.8111) -> (-102.0157, -6.6031) projected
  line L2036 (-102.0157, -6.6031) -> (-123.9275, -28.515) projected
  line L2037 (-123.9275, -28.515) -> (-102.0157, -50.4268) projected
  line L2038 (-102.0157, -50.4268) -> (-94.8078, -43.2189) projected
  line L2039 (-87.9035, -64.539) -> (-87.9035, -53.7961) projected
  line L2040 (-87.9035, -53.7961) -> (-88.0954, -53.7961) projected
  arc A205 (-94.2247, -49.82) -> (-88.0954, -53.7961) centre (-88.0954, -47.0837) ccw projected
  line L2041 (-94.2247, -49.82) -> (-98.4236, -54.0189) projected
  line L2042 (-98.4236, -54.0189) -> (-87.9035, -64.539) projected
  arc A206 (-87.9035, -85.944) -> (-87.7843, -87.2033) centre (-81.1911, -85.944) ccw projected
  line L2043 (-87.9035, -85.944) -> (-87.9035, -71.7232) projected
  line L2044 (-87.9035, -71.7232) -> (-102.0157, -57.611) projected
  line L2045 (-102.0157, -57.611) -> (-123.9275, -79.5228) projected
  line L2046 (-123.9275, -79.5228) -> (-102.0157, -101.4346) projected
  line L2047 (-102.0157, -101.4346) -> (-87.7843, -87.2033) projected
  line L2048 (81.1911, 90.2812) -> (-81.1911, 90.2812) projected
  arc A207 (-81.1911, 90.2812) -> (-84.3661, 87.1062) centre (-81.1911, 87.1062) ccw projected
  line L2049 (-84.3661, 87.1062) -> (-84.3661, 54.5958) projected
  arc A208 (-87.5411, 51.4208) -> (-84.3661, 54.5958) centre (-87.5411, 54.5958) ccw projected
  line L2050 (-87.5411, 51.4208) -> (-88.0954, 51.4208) projected
  arc A209 (-88.0954, 51.4208) -> (-91.2704, 48.2458) centre (-88.0954, 48.2458) ccw projected
  line L2051 (-91.2704, 48.2458) -> (-91.2704, -47.0837) projected
  arc A210 (-91.2704, -47.0837) -> (-88.0954, -50.2587) centre (-88.0954, -47.0837) ccw projected
  line L2052 (-88.0954, -50.2587) -> (-87.5411, -50.2587) projected
  arc A211 (-84.3661, -53.4337) -> (-87.5411, -50.2587) centre (-87.5411, -53.4337) ccw projected
  line L2053 (-84.3661, -53.4337) -> (-84.3661, -85.944) projected
  arc A212 (-84.3661, -85.944) -> (-81.1911, -89.119) centre (-81.1911, -85.944) ccw projected
  line L2054 (-81.1911, -89.119) -> (81.1911, -89.119) projected
  arc A213 (81.1911, -89.119) -> (84.3661, -85.944) centre (81.1911, -85.944) ccw projected
  line L2055 (84.3661, -85.944) -> (84.3661, -53.4337) projected
  arc A214 (87.5411, -50.2587) -> (84.3661, -53.4337) centre (87.5411, -53.4337) ccw projected
  line L2056 (87.5411, -50.2587) -> (88.0954, -50.2587) projected
  arc A215 (88.0954, -50.2587) -> (91.2704, -47.0837) centre (88.0954, -47.0837) ccw projected
  line L2057 (91.2704, -47.0837) -> (91.2704, 48.2458) projected
  arc A216 (91.2704, 48.2458) -> (88.0954, 51.4208) centre (88.0954, 48.2458) ccw projected
  line L2058 (88.0954, 51.4208) -> (87.5411, 51.4208) projected
  arc A217 (84.3661, 54.5958) -> (87.5411, 51.4208) centre (87.5411, 54.5958) ccw projected
  line L2059 (84.3661, 54.5958) -> (84.3661, 87.1062) projected
  arc A218 (84.3661, 87.1062) -> (81.1911, 90.2812) centre (81.1911, 87.1062) ccw projected